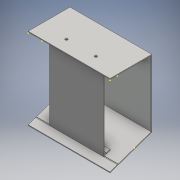
# Autodesk Inventor part: zderzaki
Saved by Autodesk Inventor 2016 (Build 200138000, 138)
## iProperties
Created: 2015-11-10
Part Number: zderzaki
Material: Ogólny
Document SubType Name: Modeling
Designer: Mrianura
Density: 1 g/cm^3
Appearance: Domyślna
Author: Mrianura
Autodesk Inventor part; units mm, degrees
ref_plane "YZ Plane" through (0, 0, 0) normal (1, 0, 0) x (0, 1, 0)
ref_plane "XZ Plane" through (0, 0, 0) normal (0, 1, 0) x (-1, 0, 0)
ref_plane "XY Plane" through (0, 0, 0) normal (0, 0, 1) x (1, 0, 0)
sketch "Szkic1" plane through (0, 0, 0) normal (1, 0, 0) x (0, 1, 0)
  line L0 (0, 0) -> (0, -88)
  line L1 (51.058, -70.4193) -> (51.058, -71.4193)
  line L2 (0, -88) -> (0, -97)
  line L3 (0, -97) -> (0, -98)
  line L4 (0, -98) -> (51.058, -80.4193)
  line L5 (51.058, -80.4193) -> (51.058, -79.4193)
  line L6 (51.058, -79.4193) -> (0, -97)
  line L7 (0, 0) -> (0, 1)
  line L8 (0, 1) -> (51.058, 1)
  line L9 (51.058, 1) -> (51.058, 2)
  line L10 (51.058, 2) -> (0, 2)
  line L11 (0, 2) -> (0, 1)
  dimension "d0" = 88
  dimension "d1" = 54
  dimension "d5" = 9
  dimension "d6" = 1
  dimension "d7" = 54
  dimension "d8" = 71
  dimension "d9" = 1
  dimension "d10" = 1
  dimension "d11" = 1
  constraints: 24 end point, 5 point on line, 3 perpendicular, 3 vertical, 1 parallel
  measures "d0" distance of L0.start L0.end
  measures "d1" distance of L0.end L1.start
  measures "d5" distance of L0.end L2.end
  measures "d6" distance of L2.end L3.end
  measures "d7" distance of L3.end L4.end
  measures "d8" angle of L4 L3
  measures "d9" distance of L4.end L5.end
  measures "d10" distance of L0.start L7.end
  measures "d11" distance of L8.end L9.end
extrude "Wyciągnięcie proste1" add sketch "Szkic1" against normal blind 100
sketch "Szkic2" plane through (-100, 0, 0) normal (-1, 0, 0) x (0, 0, 1)
  line L0 (0, 10) -> (1, 10)
  line L1 (1, 51.058) -> (1, 0) projected
  line L2 (0, 10) -> (-93.5567, 10)
  line L3 (-79.4193, 51.058) -> (-97, 0) projected
  line L4 (0, 9) -> (1, 9)
  line L5 (0, 9) -> (-93.9011, 9)
  line L6 (-93.5567, 10) -> (-93.9011, 9)
  line L7 (1, 10) -> (1, 9)
  point P0 (0, 0)
  dimension "d14" = 10
  dimension "d15" = 1
  constraints: 12 end point, 5 point on line, 2 collinear, 1 horizontal, 1 perpendicular
  measures "d14" distance of point (0, 0) L0.start
  measures "d15" distance of L0.start L4.start
extrude "Wyciągnięcie proste2" add sketch "Szkic2" against normal blind 100
sketch "Szkic3" plane through (-100, 51.058, -79.4193) normal (0, -0.3256, 0.9455) x (1, 0, 0)
  point P0 (100, -22.4199)
sketch "Szkic4" plane through (-100, 51.058, -80.4193) normal (0, 1, 0) x (1, 0, 0)
  line L0 (100, -81.4193) -> (100, 13.4817) projected
  line L1 (100, 0) -> (100, -1) projected
  line L2 (100, -81.4193) -> (100, -1)
  line L3 (0, -1) -> (0, 0) projected
  line L4 (100, -1) -> (0, -1)
  line L5 (0, 13.4817) -> (0, -81.4193) projected
  line L6 (0, -1) -> (0, -81.4193)
  line L7 (100, -81.4193) -> (0, -81.4193) projected
  line L8 (0, -81.4193) -> (100, -81.4193)
  point P0 (100, -80.4193)
  constraints: 8 end point, 3 collinear, 1 perpendicular
extrude "Wyciągnięcie proste3" add sketch "Szkic4" against normal blind 1
sketch "Szkic5" plane through (-100, 9, -93.9011) normal (0, -1, 0) x (1, 0, 0)
  point P0 (100, 93.9011)
sketch "Szkic6" plane through (-100, 51.058, -79.4193) normal (-1, 0, 0) x (0, 0, -1)
  point P0 (-79.4193, 51.058)
sketch "Szkic7" plane through (-100, 9, -93.9011) normal (0, -1, 0) x (1, 0, 0)
  line L0 (100, 14.4817) -> (100, 94.9011) projected
  line L1 (100, 94.9011) -> (90, 94.9011)
  line L2 (0, 94.9011) -> (100, 94.9011) projected
  line L3 (90, 94.9011) -> (90, 0)
  line L4 (100, 0) -> (0, 0) projected
  line L5 (90, 0) -> (100, 0)
  line L6 (100, 0) -> (100, 94.9011)
  line L7 (90, 94.9011) -> (100, 94.9011)
  line L8 (0, 94.9011) -> (10, 94.9011)
  line L9 (10, 94.9011) -> (10, 0)
  line L10 (0, 0) -> (0, 94.9011) projected
  line L11 (10, 0) -> (0, 0)
  line L12 (0, 94.9011) -> (0, 14.4817) projected
  line L13 (0, 0) -> (0, 94.9011)
  line L14 (0, 94.9011) -> (10, 94.9011)
  point P0 (100, 93.9011)
  dimension "d20" = 10
  dimension "d21" = 10
  constraints: 20 end point, 4 collinear, 4 point on line, 3 perpendicular, 1 horizontal
  measures "d20" distance of L0.end L1.end
  measures "d21" distance of L2.start L8.end
extrude "Wyciągnięcie proste4" cut sketch "Szkic7" against normal blind 1 contours L6 L4 L3 L1 L0 | L9 L4 L10 L2
sketch "Szkic8" plane through (-90, 9, 1) normal (0, -1, 0) x (1, 0, 0)
  line L0 (80, -94.9011) -> (80, 0) projected
  line L1 (80, 0) -> (73, 0)
  line L2 (80, 0) -> (0, 0) projected
  line L3 (73, 0) -> (73, -94.9011)
  line L4 (80, -94.9011) -> (0, -94.9011) projected
  line L5 (80, -94.9011) -> (80, 0)
  line L6 (90, 1) -> (-10, 1) projected
  line L7 (80, 0) -> (73, 0)
  line L8 (0, 0) -> (7, 0)
  line L9 (7, 0) -> (7, -94.9011)
  line L10 (0, -94.9011) -> (7, -94.9011)
  line L11 (0, 0) -> (0, -94.9011) projected
  line L12 (0, -94.9011) -> (0, 0)
  line L13 (0, -94.5567) -> (0, 0) projected
  point P0 (90, -1)
  dimension "d24" = 7
  dimension "d25" = 7
  constraints: 16 end point, 4 point on line, 3 collinear, 3 perpendicular
  measures "d24" distance of L0.end L1.end
  measures "d25" distance of L2.end L8.end
extrude "Wyciągnięcie proste5" cut sketch "Szkic8" against normal blind 1 contours L4 L3 L1 L0 | L4 L11 L2 L9
sketch "Szkic9" plane through (-83, 9, -93.9011) normal (-1, 0, 0) x (0, 0, 1)
  line L0 (0, 0) -> (94.9011, 0) projected
  line L1 (0, 0) -> (5, 0)
  line L2 (5, 0) -> (1.9955, 3.0045)
  line L3 (5, 0) -> (9.2489, 0) construction
  line L4 (1.9955, 3.0045) -> (1.2807, 3.7193)
  line L5 (1.2807, 3.7193) -> (2.9085, 8.4469)
  line L6 (14.4817, 42.058) -> (0.3443, 1) projected
  line L7 (2.9085, 8.4469) -> (3.854, 8.1214)
  line L8 (3.854, 8.1214) -> (2.3383, 3.7193)
  line L9 (2.3383, 3.7193) -> (5, 1)
  line L10 (94.9011, 1) -> (0.3443, 1) projected
  line L11 (5, 1) -> (5, 0)
  point P0 (93.9011, -9)
  dimension "d28" = 5
  dimension "d29" = 135
  dimension "d31" = 5
  dimension "d32" = 1
  constraints: 18 end point, 3 point on line, 2 perpendicular, 1 equal length, 1 horizontal
  measures "d28" distance of L0.start L1.end
  measures "d29" angle of L3 L2
  measures "d31" distance of L4.end L5.end
  measures "d32" distance of L5.end L7.end
extrude "Wyciągnięcie proste6" add sketch "Szkic9" against normal blind 66 contours L10 L6 L4 L2 | L2 L4 L5 L7 L8 L9 L10
sketch "Szkic10" plane through (-83, 12.7193, -91.5628) normal (0, -0.3256, 0.9455) x (1, 0, 0)
  line L0 (0.2651, 0) -> (15.2651, 0)
  line L1 (0, 0) -> (66, 0) projected
  line L2 (15.2651, 0) -> (15.2651, 2)
  line L3 (0, 4.6557) -> (66, 4.6557) projected
  circle A0 centre (15.2651, 2) radius 1.5
  line L4 (66, 0) -> (51, 0)
  line L5 (51, 0) -> (51, 2)
  circle A1 centre (51, 2) radius 1.5
  point P0 (83, 17.7836)
  dimension "d35" = 15
  dimension "d36" = 2
  dimension "d37" = 3
  dimension "d38" = 15
  dimension "d39" = 2
  dimension "d40" = 3
  constraints: 8 end point, 2 centre point, 2 coincident, 2 perpendicular, 2 point on line
  measures "d35" distance of L0.start L0.end
  measures "d36" distance of L0.end L2.end
  measures "d37" diameter of A0
  measures "d38" distance of L1.end L4.end
  measures "d39" distance of L4.end L5.end
  measures "d40" diameter of A1
extrude "Wyciągnięcie proste7" cut sketch "Szkic10" against normal blind 15
sketch "Szkic11" plane through (-83, 9, -93.9011) normal (-1, 0, 0) x (0, 0, 1)
  line L0 (94.9011, 1) -> (5, 1) projected
  line L1 (94.9011, 1) -> (90.2011, 1)
  line L2 (90.2011, 1) -> (93.0515, 3.8505)
  line L3 (93.0515, 3.8505) -> (94.9011, 5.7)
  line L4 (94.9011, 41.058) -> (94.9011, -9) projected
  line L5 (90.2011, 1) -> (89.2011, 1)
  line L6 (94.9011, 0) -> (94.9011, 1) projected
  line L7 (94.9011, 1) -> (94.9011, 9)
  line L8 (94.9011, 9) -> (93.9011, 9)
  line L9 (93.9011, 9) -> (93.9011, 5.7)
  line L10 (93.9011, 5.7) -> (89.2011, 1)
  line L11 (94.9011, 9) -> (94.9011, 5.7)
  point P0 (93.9011, -9)
  dimension "d43" = 4.7
  dimension "d44" = 45
  dimension "d45" = 1
  dimension "d46" = 8
  dimension "d47" = 1
  constraints: 18 end point, 5 point on line, 2 perpendicular, 1 collinear
  measures "d43" distance of L0.start L1.end
  measures "d44" angle of L1 L2
  measures "d45" distance of L1.end L5.end
  measures "d46" distance of L0.start L7.end
  measures "d47" distance of L7.end L8.end
extrude "Wyciągnięcie proste8" add sketch "Szkic11" against normal blind 66
sketch "Szkic12" plane through (-83, 14.7, 0) normal (0, 0, -1) x (-1, 0, 0)
  point P0 (-83, -14.7)
sketch "Szkic13" plane through (-83, 9, -93.9011) normal (-1, 0, 0) x (0, 0, 1)
  line L0 (93.9011, 5.7) -> (89.2011, 1) projected
  line L1 (89.2011, 1) -> (91.885, 2.5496)
  line L2 (89.2011, 1) -> (92.3002, 1) construction
  line L3 (91.885, 2.5496) -> (93.9011, 3.7135)
  line L4 (93.9011, 5.7) -> (93.9011, 3.7135)
  line L5 (5, 1) -> (89.2011, 1) projected
  line L6 (93.9011, 5.7) -> (89.2011, 1)
  point P0 (93.9011, -9)
  dimension "d50" = 30
  constraints: 10 end point, 1 collinear, 1 equal length, 1 horizontal, 1 perpendicular, 1 point on line
  measures "d50" angle of L2 L1
extrude "Wyciągnięcie proste9" cut sketch "Szkic13" against normal blind 66
sketch "Szkic14" plane through (-17, 18, 0) normal (0, 0, -1) x (-1, 0, 0)
  line L0 (66, -5.2865) -> (0, -5.2865) projected
  line L1 (66, -5.2865) -> (51, -5.2865)
  line L2 (51, -5.2865) -> (51, -3.2865)
  circle A0 centre (51, -3.2865) radius 1.5
  line L3 (0, -5.2865) -> (0, 0) projected
  line L4 (0, -5.2865) -> (15, -5.2865)
  line L5 (15, -5.2865) -> (15, -3.2865)
  circle A1 centre (15, -3.2865) radius 1.5
  point P0 (-17, -18)
  dimension "d53" = 15
  dimension "d54" = 2
  dimension "d55" = 3
  dimension "d56" = 15
  dimension "d57" = 2
  dimension "d58" = 3
  constraints: 8 end point, 2 centre point, 2 coincident, 2 perpendicular, 2 point on line
  measures "d53" distance of L0.start L1.end
  measures "d54" distance of L1.end L2.end
  measures "d55" diameter of A0
  measures "d56" distance of L0.end L4.end
  measures "d57" distance of L4.end L5.end
  measures "d58" diameter of A1
extrude "Wyciągnięcie proste10" cut sketch "Szkic14" against normal blind 15
sketch "Szkic15" plane through (-83, 9, -93.9011) normal (-1, 0, 0) x (0, 0, 1)
  point P0 (93.9011, -9)
sketch "Szkic16" plane through (-17, 18, 0) normal (0, 0, -1) x (-1, 0, 0)
  point P0 (-17, -18)
sketch "Szkic17" plane through (-83, 9, -93.9011) normal (-1, 0, 0) x (0, 0, 1)
  line L0 (94.9011, 9) -> (93.9011, 9) projected
  line L1 (94.9011, 9) -> (94.9011, 8)
  line L2 (94.9011, 41.058) -> (94.9011, -9) projected
  line L3 (94.9011, 8) -> (93.9011, 8)
  line L4 (93.9011, 3.7135) -> (93.9011, 9) projected
  line L5 (93.9011, 9) -> (94.9011, 9)
  point P0 (93.9011, -9)
  dimension "d61" = 1
  constraints: 6 end point, 2 point on line, 1 collinear, 1 perpendicular
  measures "d61" distance of L0.start L1.end
extrude "Wyciągnięcie proste11" cut sketch "Szkic17" against normal blind 66
